Autodesk Inventor part; units mm, degrees
(part 2 of 2)
extrude "Extrusion1" add sketch "Sketch1" along normal blind 1.5 contours L99 A73 A72 L100 A81 A82 L118 A78 L121 A84 L120 A83 L116 A79 L117 A80 L126 A93 L127 A89 L128 A90 L129 A92 A91 L101 A95 A94 L107 A77 L114 A76 L113 A75 L112 A74 | L107 A85 L122 A88 L124 A87 L123 A86 | L363 A265 A264 L364 A273 A274 L382 A270 L385 A276 L384 A275 L380 A271 L381 A272 L390 A285 L391 A281 L392 A282 L393 A284 A283 L365 A287 A286 L371 A269 L378 A268 L377 A267 L376 A266 | L371 A277 L386 A280 L388 A279 L387 A278 | L403 L402 L397 L405
sketch "Sketch4" plane through (0, 1.5, 0) normal (0, 1, 0) x (1, 0, 0)
  line L0 (-3.25, -8.45) -> (-5.75, -8.45) construction
  line L1 (-7.25, -5.8376) -> (-7.25, 5.8376) construction
  arc A0 (45.25, -7.25) -> (45.4265, -6.0765) centre (45.25, -6.65) ccw construction
  line L2 (64.25, 24.8376) -> (64.25, 13.1624) construction
  line L3 (62.75, 10.55) -> (60.25, 10.55) construction
  line L4 (-5.75, 46.45) -> (-3.25, 46.45) construction
  line L5 (-9.25, -9.25) -> (66.25, -9.25)
  line L6 (66.25, -9.25) -> (66.25, 47.25)
  line L7 (66.25, 47.25) -> (-9.25, 47.25)
  line L8 (-9.25, 47.25) -> (-9.25, -9.25)
  line L9 (66.25, -9.25) -> (47.8433, -9.25)
  line L10 (47.8433, -9.25) -> (47.8433, 9.75)
  line L11 (47.8433, 9.75) -> (66.25, 9.75)
  line L12 (66.25, 9.75) -> (66.25, -9.25)
  line L13 (66.25, 19) -> (62.176, 19)
  line L14 (47.8433, 47.25) -> (47.8433, 28.25)
  line L15 (47.8433, 28.25) -> (66.25, 28.25)
  line L16 (76.5, -18.5) -> (-38.5, -18.5)
  line L17 (-38.5, -18.5) -> (-38.5, 56.5)
  line L18 (-38.5, 56.5) -> (76.5, 56.5)
  line L19 (76.5, 56.5) -> (76.5, -18.5)
  line L20 (2.65, -7.25) -> (-2.65, -7.25) construction
  line L21 (59.65, 11.75) -> (54.35, 11.75) construction
  line L22 (-38.5, 52.5) -> (-38.5, -14.5) construction
  line L23 (71.52, -14.5) -> (-38.5, -14.5)
  line L24 (-38.5, -14.5) -> (-38.5, 52.5)
  line L25 (-38.5, 52.5) -> (71.52, 52.5)
  line L26 (71.52, 52.5) -> (71.52, -14.5)
  point P0 (0, 0)
  point P1 (-4.5, -8.45)
  point P2 (-4.5, 46.45)
  point P3 (45.8433, -6.7392)
  point P4 (61.5, 10.55)
  point P5 (47.8433, -9.25)
  point P6 (-38.5, -18.5)
  dimension "d38" = 2
  dimension "d40" = 2
  dimension "d41" = 2
  dimension "d79" = 2
  dimension "d80" = 2
  dimension "d81" = 29.25
  constraints: 38 end point, 8 parallel, 5 horizontal, 4 midpoint, 4 perpendicular, 3 symmetric about line, 1 point on circle
  measures "d38" distance between parallel lines of L1 L8
  measures "d40" distance from line of L13.start L2
  measures "d41" distance from line of L10 point (45.843, -6.739)
  measures "d79" distance between parallel lines of L5 L20
  measures "d80" distance between parallel lines of L11 L21
  measures "d81" distance between parallel lines of L8 L22
extrude "Extrusion6" add sketch "Sketch4" along normal blind 6 contours L10 L11 L6 L5 | L7 L6 L15 L14 | L17 L25 L26 L23
ref_plane "Work Plane3" through (-9.25, 7.5, 9.25) normal (-0.7071068, -0.7071068, 0) x (0, 0, -1)
sketch "Sketch6" plane through (-9.25, 7.5, 9.25) normal (-0.7071068, -0.7071068, 0) x (0, 0, -1)
  line L0 (0, 0) -> (56.5, 0) construction
  line L1 (-4.25, 0) -> (26.75, 0)
  line L2 (26.75, 0) -> (26.75, -30)
  line L3 (26.75, -30) -> (-4.25, -30)
  line L4 (-4.25, -30) -> (-4.25, 0)
  line L5 (-9.25, -20.6829) -> (-9.25, 60.6344) construction
  point P0 (9.25, 11.844)
  dimension "d48" = 31
  dimension "d49" = 30
  dimension "d50" = 5
  constraints: 8 end point, 2 parallel, 1 horizontal, 1 perpendicular, 1 point on line
  measures "d48" distance of L2.end L3.end
  measures "d49" distance of L1.end L2.end
  measures "d50" distance between parallel lines of L5 L4
sketch "Sketch7" plane through (0, 7.5, 0) normal (0, 1, 0) x (1, 0, 0)
  line L0 (-38.5, 52.5) -> (-38.5, -14.5) construction
  line L1 (-9.25, -9.25) -> (-38.5, -9.25)
  line L2 (-38.5, -9.25) -> (-38.5, 22.75)
  line L3 (-38.5, 22.75) -> (-9.25, 22.75)
  line L4 (-9.25, 22.75) -> (-9.25, -9.25)
  point P0 (-38.5, 56.5)
  point P1 (-38.5, -18.5)
  point P2 (0, 0)
  dimension "d51" = 32
  constraints: 8 end point, 2 parallel, 1 horizontal, 1 perpendicular, 1 point on line
  measures "d51" distance of L1.end L2.end
extrude "Extrusion7" add sketch "Sketch7" along normal blind 7
sketch "Sketch8" plane through (-38.5, 7.5, 9.25) normal (0, 0, 1) x (1, 0, 0)
  line L0 (0, 7) -> (29.25, 7) construction
  line L1 (29.25, 7) -> (4, 26.658)
  line L2 (0, 7) -> (0, 45.8303)
  line L3 (4, 26.658) -> (0, 26.658)
  line L4 (0, 7) -> (29.25, 7)
  point P0 (38.5, -7.5)
  dimension "d54" = 32
  dimension "d55" = 4
  dimension "d56" = 37.902
  constraints: 8 end point, 1 perpendicular, 1 point on line, 1 vertical
  measures "d54" distance of L0.end L1.end
  measures "d55" distance of L3.end L1.end
  measures "d56" angle of L1 L0
extrude "Extrusion8" add sketch "Sketch8" against normal up to surface (32 mm away)
sketch "Sketch9" plane through (-38.5, 7.5, 9.25) normal (0, 0, 1) x (1, 0, 0)
  line L0 (29.25, 0) -> (0, 0) construction
  line L1 (29.25, 0) -> (29.25, 7) construction
  line L2 (29.25, 7) -> (4, 26.658) construction
  line L3 (4, 26.658) -> (0, 26.658) construction
  line L4 (0, 0) -> (0, 26.658) construction
  line L5 (0, 24.658) -> (4.1272, 24.658)
  line L6 (4.1272, 24.658) -> (27.25, 6.6561)
  line L7 (27.25, 6.6561) -> (27.25, 0)
  line L8 (27.25, 0) -> (27.25, -7.5)
  line L9 (0, -7.5) -> (115, -7.5) construction
  line L10 (27.25, -7.5) -> (0, -7.5)
  line L11 (0, -7.5) -> (0, 24.658)
  point P0 (38.5, -7.5)
  point P1 (27.25, 0)
  dimension "d60" = 1.5
  dimension "d61" = 2
  dimension "d62" = 2
  constraints: 12 end point, 3 perpendicular, 2 point on line, 1 horizontal, 1 parallel, 1 vertical, 1 other
  measures "d60" distance between parallel lines of L6 L2
  measures "d61" distance between parallel lines of L5 L3
ref_plane "Work Plane4" through (-38.5, 7.5, 7.25) normal (0, 0, 1) x (1, 0, 0)
extrude "Extrusion9" cut sketch "Sketch9" against normal blind 28 from surface at -2
sketch "Sketch10" plane through (-34.3728, 32.158, -20.75) normal (-0.6143129, -0.7890625, 0) x (0, 0, 1)
  line L0 (28, 0) -> (28, -29.3042) construction
  line L1 (0, 0) -> (28, 0) construction
  line L2 (0, 0) -> (0, -29.3042) construction
  line L3 (0, -29.3042) -> (28, -29.3042) construction
  line L4 (2.5, -26.1712) -> (25.5, -26.1712) construction
  line L5 (25.5, -26.1712) -> (25.5, -3.1712) construction
  line L6 (25.5, -3.1712) -> (2.5, -3.1712) construction
  line L7 (2.5, -3.1712) -> (2.5, -26.1712) construction
  line L8 (2.5, -26.1712) -> (25.5, -3.1712) construction
  line L9 (25.5, -26.1712) -> (2.5, -3.1712) construction
  circle A0 centre (2.5, -3.1712) radius 0.75
  circle A1 centre (25.5, -3.1712) radius 0.75
  circle A2 centre (25.5, -26.1712) radius 0.75
  circle A3 centre (2.5, -26.1712) radius 0.75
  line L10 (1, -5.1712) -> (27, -5.1712)
  line L11 (27, -5.1712) -> (27, -22.6712)
  line L12 (27, -22.6712) -> (1, -22.6712)
  line L13 (1, -22.6712) -> (1, -5.1712)
  line L14 (1, -5.1712) -> (27, -22.6712) construction
  line L15 (27, -5.1712) -> (1, -22.6712) construction
  point P0 (20.75, -46.8774)
  point P1 (14, -14.6712)
  point P2 (14, -13.9212)
  dimension "d66" = 29.3042
  dimension "d67" = 28
  dimension "d68" = 23
  dimension "d69" = 23
  dimension "d70" = 1.5
  dimension "d71" = 1.5
  dimension "d72" = 0.75
  dimension "d73" = 17.5
  dimension "d74" = 26
  constraints: 24 end point, 4 centre point, 4 midpoint, 4 parallel, 2 coincident, 2 horizontal, 2 perpendicular, 2 symmetric about line, 2 other
  measures "d66" distance between parallel lines of L3 L1
  measures "d67" distance between parallel lines of L2 L0
  measures "d68" distance of L6.end L5.end
  measures "d69" distance of L5.end L4.end
  measures "d70" diameter of A0
  measures "d71" diameter of A1
  measures "d72" distance of point (14, -14.671) point (14, -13.921)
  measures "d73" distance of L11.end L10.end
  measures "d74" distance of L11.end L12.end
extrude "Extrusion10" cut sketch "Sketch10" against normal through all contours L10 L11 L12 L13
extrude "Extrusion11" add sketch "Sketch10" along normal blind 5 contours A0 | A1 | A2 | A3
fillet "Fillet1" radius 1 8 edges at (-9.25, 4.5, -47.25) (47.8433, 4.5, -47.25) (47.8433, 4.5, -28.25) (66.25, 4.5, -28.25) (66.25, 4.5, -9.75) (47.8433, 4.5, -9.75) (47.8433, 4.5, 9.25) (-9.25, 4.5, 9.25)
fillet "Fillet2" radius 5 4 edges at (71.52, 3.75, -52.5) (71.52, 3.75, 14.5) (-38.5, 3.75, -52.5) (-38.5, 3.75, 14.5)
sketch "Sketch11" plane through (0, 7.5, 0) normal (0, 1, 0) x (1, 0, 0)
  circle A0 centre (-23.5, 37.75) radius 3.625
  line L0 (-38.5, 47.5) -> (-38.5, 22.75) construction
  line L1 (-38.5, 22.75) -> (-9.25, 22.75) construction
  point P0 (0, 0)
  dimension "d86" = 7.25
  dimension "d89" = 15
  dimension "d90" = 15
  constraints: 1 centre point
  measures "d86" diameter of A0
  measures "d89" distance from line of L1 A0.centre
  measures "d90" distance from line of L0 A0.centre
extrude "Extrusion12" cut sketch "Sketch11" against normal through all
sketch "Sketch12" plane through (0, 0, 0) normal (0, -1, 0) x (1, 0, 0)
  line L0 (-33.5, 14.5) -> (66.52, 14.5) construction
  line L1 (-30.25, 14.5) -> (9.75, 14.5)
  line L2 (9.75, 14.5) -> (9.75, 11.5)
  line L3 (9.75, 11.5) -> (-30.25, 11.5)
  line L4 (-30.25, 11.5) -> (-30.25, 14.5)
  point P0 (-38.5, 9.5)
  point P1 (0, 0)
  point P2 (-30.25, 13)
  dimension "d91" = 3
  dimension "d92" = 8.25
  dimension "d93" = 40
  constraints: 8 end point, 2 parallel, 1 horizontal, 1 midpoint, 1 perpendicular, 1 point on line
  measures "d91" distance of L1.end L2.end
  measures "d92" horizontal distance of point (-38.5, 9.5) point (-30.25, 13)
  measures "d93" distance of L2.end L3.end
extrude "Extrusion13" cut sketch "Sketch12" against normal blind 2
sketch "Sketch13" plane through (0, 0, 0) normal (0, -1, 0) x (1, 0, 0)
  circle A0 centre (-34.5, 10.5) radius 2
  line L0 (-33.5, 14.5) -> (-30.25, 14.5) projected
  line L1 (-38.5, 7.25) -> (-38.5, 9.5) projected
  line L2 (66.52, -52.5) -> (-33.5, -52.5) construction
  line L3 (16.51, -52.5) -> (16.51, 14.5) construction
  line L4 (9.75, 14.5) -> (66.52, 14.5) construction
  line L5 (71.52, 9.5) -> (71.52, -47.5) construction
  line L6 (71.52, -19) -> (-38.5, -19) construction
  line L7 (-38.5, -20.75) -> (-38.5, 7.25) construction
  circle A1 centre (67.52, 10.5) radius 2
  circle A2 centre (-34.5, -48.5) radius 2
  circle A3 centre (67.52, -48.5) radius 2
  point P0 (0, 0)
  dimension "d96" = 4
  dimension "d97" = 4
  dimension "d98" = 4
  constraints: 4 centre point, 4 end point, 3 symmetric about line, 2 midpoint, 2 point on line, 1 horizontal, 1 vertical, 3 other
  measures "d96" diameter of A0
  measures "d97" distance from line of L0 A0.centre
  measures "d98" distance from line of L1 A0.centre
extrude "Extrusion14" cut sketch "Sketch13" against normal blind 5
body "Solid1"
